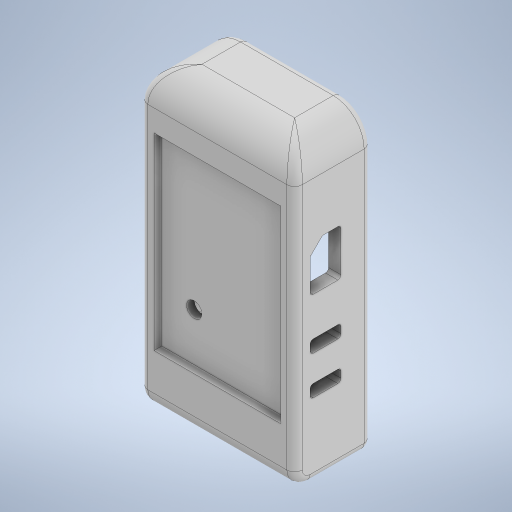
# Autodesk Inventor part: Součást1
Saved by Autodesk Inventor 2024 (Build 280153000, 153)
## iProperties
Created: 2024-02-27
Part Number: Součást1
Material: Všeobecné
Document SubType Name: Modeling
Designer: zak
Density: 1 g/cm^3
Appearance: Výchozí
Author: zak
Autodesk Inventor part; units mm, degrees
ref_plane "YZ Plane" through (0, 0, 0) normal (1, 0, 0) x (0, 1, 0)
ref_plane "XZ Plane" through (0, 0, 0) normal (0, 1, 0) x (-1, 0, 0)
ref_plane "XY Plane" through (0, 0, 0) normal (0, 0, 1) x (1, 0, 0)
sketch "Náčrt1" plane through (0, 0, 0) normal (0, 0, 1) x (1, 0, 0)
  line L0 (-50, -95) -> (50, -95)
  line L1 (50, -95) -> (50, 95)
  line L2 (50, 95) -> (-50, 95)
  line L3 (-50, 95) -> (-50, -95)
  line L4 (-50, -95) -> (50, 95) construction
  line L5 (50, -95) -> (-50, 95) construction
  point P0 (0, 0)
  dimension "d0" = 100
  dimension "d1" = 190
  constraints: 12 end point, 2 midpoint, 2 parallel, 1 horizontal, 1 perpendicular
  measures "d0" distance of L2.end L1.end
  measures "d1" distance of L1.end L0.end
extrude "Vysunutí1" add sketch "Náčrt1" along normal blind 50
sketch "Náčrt2" plane through (0, 0, 0) normal (0, 0, -1) x (-1, 0, 0)
  point P0 (0, 0)
sketch "Náčrt4" plane through (0, 0, 0) normal (0, 0, -1) x (-1, 0, 0)
  line L0 (42, 45) -> (-42, 45)
  line L1 (-42, 45) -> (-42, -65)
  line L2 (-42, -65) -> (42, -65)
  line L3 (42, -65) -> (42, 45)
  line L4 (42, 45) -> (-42, -65) construction
  line L5 (-42, 45) -> (42, -65) construction
  point P0 (0, 0)
  point P1 (0, -10)
  dimension "d8" = 84
  dimension "d9" = 110
  constraints: 12 end point, 2 midpoint, 2 parallel, 1 horizontal, 1 perpendicular
  measures "d8" distance of L2.end L1.end
  measures "d9" distance of L1.end L0.end
extrude "Vysunutí3" cut sketch "Náčrt4" against normal blind 40
fillet "Zaoblení1" radius 20 3 edges at (0, 95, 50) (-50, 95, 25) (50, 95, 25)
fillet "Zaoblení2" radius 10 1 edges at (0, -95, 50)
sketch "Náčrt5" plane through (0, 0, 40) normal (0, 0, -1) x (-1, 0, 0)
  circle A0 centre (37, 40) radius 5
  line L0 (42, 45) -> (42, -65) projected
  line L1 (-42, 45) -> (42, 45) projected
  circle A1 centre (37, -60) radius 5
  circle A2 centre (-37, 40) radius 5
  circle A3 centre (-37, -60) radius 5
  line L2 (42, 45) -> (32, 45)
  line L3 (32, 45) -> (32, 35)
  line L4 (32, 35) -> (42, 35)
  line L5 (42, 35) -> (42, 45)
  line L6 (42, 45) -> (32, 35) construction
  line L7 (32, 45) -> (42, 35) construction
  line L8 (42, -65) -> (32, -65)
  line L9 (32, -65) -> (32, -55)
  line L10 (32, -55) -> (42, -55)
  line L11 (42, -55) -> (42, -65)
  line L12 (42, -65) -> (32, -55) construction
  line L13 (32, -65) -> (42, -55) construction
  line L14 (-42, -65) -> (-32, -65)
  line L15 (-32, -65) -> (-32, -55)
  line L16 (-32, -55) -> (-42, -55)
  line L17 (-42, -55) -> (-42, -65)
  line L18 (-42, -65) -> (-32, -55) construction
  line L19 (-32, -65) -> (-42, -55) construction
  line L20 (-32, 45) -> (-42, 45)
  line L21 (-42, 45) -> (-42, 35)
  line L22 (-42, 35) -> (-32, 35)
  line L23 (-32, 35) -> (-32, 45)
  line L24 (-32, 45) -> (-42, 35) construction
  line L25 (-42, 45) -> (-32, 35) construction
  line L26 (42, 45) -> (32, 45)
  line L27 (32, 45) -> (32, 35)
  line L28 (32, 35) -> (42, 35)
  line L29 (42, 35) -> (42, 45)
  line L30 (42, 45) -> (32, 35) construction
  line L31 (32, 45) -> (42, 35) construction
  line L32 (32, -55) -> (32, -65)
  line L33 (32, -65) -> (42, -65)
  line L34 (42, -65) -> (42, -55)
  line L35 (42, -55) -> (32, -55)
  line L36 (-42, 45) -> (-42, 35)
  line L37 (-42, 35) -> (-32, 35)
  line L38 (-32, 35) -> (-32, 45)
  line L39 (-32, 45) -> (-42, 45)
  line L40 (-42, -55) -> (-42, -65)
  line L41 (-42, -65) -> (-32, -65)
  line L42 (-32, -65) -> (-32, -55)
  line L43 (-32, -55) -> (-42, -55)
  point P0 (0, 0)
  point P1 (32, -155)
  point P2 (-116, 35)
  point P3 (-42, -155)
  point P4 (-116, -65)
  point P5 (-32, 40)
  point P6 (-37, 35)
  point P7 (-37, 45)
  point P8 (-42, 40)
  point P9 (-42, -60)
  point P10 (-37, -55)
  point P11 (-37, -65)
  point P12 (-32, -60)
  point P13 (37, -65)
  point P14 (42, -60)
  point P15 (32, -60)
  point P16 (37, -55)
  point P17 (37, 45)
  point P18 (42, 40)
  point P19 (32, 40)
  point P20 (37, 35)
  dimension "d16" = 100
  dimension "d19" = 74
  dimension "d143" = 100
  dimension "d146" = 74
  constraints: 84 end point, 10 midpoint, 10 parallel, 10 point on line, 7 horizontal, 5 perpendicular, 4 centre point, 2 vertical, 1 tangent, 36 other
  measures "d16" distance of A0.centre A1.centre
  measures "d19" distance of A0.centre A2.centre
  measures "d143" distance of L2.end L32.start
  measures "d146" distance of L2.end L36.start
extrude "Vysunutí4" add sketch "Náčrt5" along normal blind 40
sketch "Náčrt6" plane through (0, 0, 0) normal (0, 0, -1) x (-1, 0, 0)
  arc A0 (37, 45) -> (42, 40) centre (37, 40) ccw projected
  circle A1 centre (37, 40) radius 2.5
  circle A2 centre (-37, 40) radius 2.5
  arc A3 (-37, -65) -> (-42, -60) centre (-37, -60) ccw projected
  circle A4 centre (-37, -60) radius 2.5
  arc A5 (42, -60) -> (37, -65) centre (37, -60) ccw projected
  circle A6 centre (37, -60) radius 2.5
  point P0 (0, 0)
  dimension "d24" = 5
  dimension "d25" = 5
  dimension "d26" = 5
  dimension "d27" = 5
  constraints: 4 centre point, 3 coincident
  measures "d24" diameter of A1
  measures "d25" diameter of A2
  measures "d26" diameter of A4
  measures "d27" diameter of A6
extrude "Vysunutí5" cut sketch "Náčrt6" against normal blind 10
sketch "Náčrt9" plane through (-37, -65, 0) normal (0, 1, 0) x (1, 0, 0)
  line L0 (30.5, -29) -> (43.5, -29)
  line L1 (43.5, -29) -> (43.5, -11)
  line L2 (43.5, -11) -> (30.5, -11)
  line L3 (30.5, -11) -> (30.5, -29)
  line L4 (30.5, -29) -> (43.5, -11) construction
  line L5 (43.5, -29) -> (30.5, -11) construction
  circle A0 centre (30.5, -11) radius 1.75
  circle A1 centre (43.5, -11) radius 1.75
  circle A2 centre (43.5, -29) radius 1.75
  circle A3 centre (30.5, -29) radius 1.75
  circle A4 centre (30.5, -29) radius 1
  circle A5 centre (30.5, -11) radius 1
  circle A6 centre (43.5, -11) radius 1
  circle A7 centre (43.5, -29) radius 1
  point P0 (37, 0)
  point P1 (37, -20)
  dimension "d30" = 13
  dimension "d31" = 18
  dimension "d32" = 3.5
  dimension "d33" = 3.5
  dimension "d34" = 3.5
  dimension "d35" = 3.5
  dimension "d128" = 2
  dimension "d129" = 2
  dimension "d130" = 2
  dimension "d131" = 2
  constraints: 12 end point, 8 centre point, 7 coincident, 2 midpoint, 2 parallel, 1 horizontal, 1 perpendicular, 1 point on line
  measures "d30" distance of L2.end L1.end
  measures "d31" distance of L1.end L0.end
  measures "d32" diameter of A0
  measures "d33" diameter of A1
  measures "d34" diameter of A2
  measures "d35" diameter of A3
  measures "d128" diameter of A4
  measures "d129" diameter of A5
  measures "d130" diameter of A6
  measures "d131" diameter of A7
extrude "Vysunutí6" add sketch "Náčrt9" along normal blind 4 contours A4 L3 A3 L0 | L0 A3 L3 A4 | A2 L1 A7 L0 | L0 A7 L1 A2 | A0 L2 A5 L3 | L3 A5 L2 A0 | A1 L2 A6 L1 | L1 A6 L2 A1
sketch "Náčrt11" plane through (-37, 45, 0) normal (0, -1, 0) x (1, 0, 0)
  line L0 (30.5, 11) -> (43.5, 11)
  line L1 (43.5, 11) -> (43.5, 29)
  line L2 (43.5, 29) -> (30.5, 29)
  line L3 (30.5, 29) -> (30.5, 11)
  line L4 (30.5, 11) -> (43.5, 29) construction
  line L5 (43.5, 11) -> (30.5, 29) construction
  circle A0 centre (30.5, 11) radius 1.75
  circle A1 centre (30.5, 29) radius 1.75
  circle A2 centre (43.5, 11) radius 1.75
  circle A3 centre (43.5, 29) radius 1.75
  circle A4 centre (30.5, 11) radius 1
  circle A5 centre (30.5, 29) radius 1
  circle A6 centre (43.5, 11) radius 1
  circle A7 centre (43.5, 29) radius 1
  point P0 (37, 0)
  point P1 (37, 20)
  dimension "d49" = 13
  dimension "d50" = 18
  dimension "d51" = 3.5
  dimension "d52" = 3.5
  dimension "d53" = 3.5
  dimension "d54" = 3.5
  dimension "d132" = 2
  dimension "d135" = 18
  dimension "d138" = 13
  constraints: 12 end point, 8 centre point, 5 coincident, 2 horizontal, 2 midpoint, 2 parallel, 1 perpendicular, 1 vertical, 6 other
  measures "d49" distance of L2.end L1.end
  measures "d50" distance of L1.end L0.end
  measures "d51" diameter of A0
  measures "d52" diameter of A1
  measures "d53" diameter of A2
  measures "d54" diameter of A3
  measures "d132" diameter of A4
  measures "d135" distance of A4.centre A5.centre
  measures "d138" distance of A4.centre A6.centre
extrude "Vysunutí8" add sketch "Náčrt11" along normal blind 4 contours A4 L3 A0 L0 | L0 A0 L3 A4 | A2 L1 A6 L0 | L0 A6 L1 A2 | A1 L2 A5 L3 | L3 A5 L2 A1 | A3 L2 A7 L1 | L1 A7 L2 A3
fillet "Zaoblení3" radius 5 8 edges at (-50, -92.0711, 47.0711) (-50, -95, 20) (-44.1421, 89.1421, 44.1421) (-50, -5, 50) (44.1421, 89.1421, 44.1421) (50, -92.0711, 47.0711) (50, -95, 20) (50, -5, 50)
fillet "Zaoblení4" radius 5 8 edges at (-44.1421, 89.1421, 0) (-50, -7.5, 0) (-48.5355, -93.5355, 0) (0, -95, 0) (48.5355, -93.5355, 0) (50, -7.5, 0) (44.1421, 89.1421, 0) (0, 95, 0)
sketch "Náčrt17" plane through (0, 0, 0) normal (0, 0, -1) x (-1, 0, 0)
  line L0 (38.0929, 83.7446) -> (-38.0929, 83.7446)
  line L1 (-40.0929, 81.7446) -> (-40.0929, 58.2554)
  line L2 (-38.0929, 56.2554) -> (38.0929, 56.2554)
  line L3 (40.0929, 58.2554) -> (40.0929, 81.7446)
  line L4 (40.0929, 83.7446) -> (-40.0929, 56.2554) construction
  line L5 (-40.0929, 83.7446) -> (40.0929, 56.2554) construction
  arc A0 (40.0929, 81.7446) -> (38.0929, 83.7446) centre (38.0929, 81.7446) ccw
  arc A1 (38.0929, 56.2554) -> (40.0929, 58.2554) centre (38.0929, 58.2554) ccw
  arc A2 (-40.0929, 58.2554) -> (-38.0929, 56.2554) centre (-38.0929, 58.2554) ccw
  arc A3 (-38.0929, 83.7446) -> (-40.0929, 81.7446) centre (-38.0929, 81.7446) ccw
  line L6 (40, -87.5) -> (-40, -87.5)
  line L7 (-42, -85.5) -> (-42, -74.5)
  line L8 (-40, -72.5) -> (40, -72.5)
  line L9 (42, -74.5) -> (42, -85.5)
  line L10 (42, -87.5) -> (-42, -72.5) construction
  line L11 (-42, -87.5) -> (42, -72.5) construction
  arc A4 (40, -87.5) -> (42, -85.5) centre (40, -85.5) ccw
  arc A5 (42, -74.5) -> (40, -72.5) centre (40, -74.5) ccw
  arc A6 (-40, -72.5) -> (-42, -74.5) centre (-40, -74.5) ccw
  arc A7 (-42, -85.5) -> (-40, -87.5) centre (-40, -85.5) ccw
  point P0 (0, 0)
  point P1 (0, 70)
  point P2 (0, -80)
  dimension "d82" = 2
  dimension "d83" = 15
  dimension "d84" = 2
  constraints: 24 end point, 16 point on circle, 16 point on line, 16 tangent, 8 centre point, 6 equal radius, 4 midpoint, 4 parallel, 2 horizontal, 2 perpendicular
  measures "d82" radius of A0
  measures "d83" distance of L11.start L10.end
  measures "d84" radius of A4
extrude "Vysunutí12" cut sketch "Náčrt17" against normal blind 35
sketch "Náčrt18" plane through (0, 0, 50) normal (0, 0, 1) x (1, 0, 0)
  line L0 (41, 61) -> (-41, 61)
  line L1 (-41, 61) -> (-41, -61)
  line L2 (-41, -61) -> (41, -61)
  line L3 (41, -61) -> (41, 61)
  line L4 (41, 61) -> (-41, -61) construction
  line L5 (-41, 61) -> (41, -61) construction
  point P0 (0, 0)
  dimension "d87" = 82
  dimension "d88" = 122
  constraints: 12 end point, 2 midpoint, 2 parallel, 1 horizontal, 1 perpendicular
  measures "d87" distance of L2.end L1.end
  measures "d88" distance of L1.end L0.end
extrude "Vysunutí13" cut sketch "Náčrt18" against normal blind 5
sketch "Náčrt20" plane through (-50, -85, 45) normal (-1, 0, 0) x (0, 0, 1)
  line L0 (-5, 120) -> (-5, 30) projected
  line L1 (-13.8284, 125) -> (-23, 125)
  line L2 (-25, 123) -> (-25, 97)
  line L3 (-23, 95) -> (-7, 95)
  line L4 (-5, 97) -> (-5, 116.1716)
  line L5 (-5.5858, 117.5858) -> (-12.4142, 124.4142)
  arc A0 (-23, 125) -> (-25, 123) centre (-23, 123) ccw
  arc A1 (-12.4142, 124.4142) -> (-13.8284, 125) centre (-13.8284, 123) ccw
  arc A2 (-5, 116.1716) -> (-5.5858, 117.5858) centre (-7, 116.1716) ccw
  arc A3 (-7, 95) -> (-5, 97) centre (-7, 97) ccw
  arc A4 (-25, 97) -> (-23, 95) centre (-23, 97) ccw
  line L6 (-7, 70) -> (-23, 70)
  line L7 (-25, 68) -> (-25, 64)
  line L8 (-23, 62) -> (-7, 62)
  line L9 (-5, 64) -> (-5, 68)
  line L10 (-7, 45) -> (-23, 45)
  line L11 (-25, 43) -> (-25, 39)
  line L12 (-23, 37) -> (-7, 37)
  line L13 (-5, 39) -> (-5, 43)
  arc A5 (-5, 68) -> (-7, 70) centre (-7, 68) ccw
  arc A6 (-7, 62) -> (-5, 64) centre (-7, 64) ccw
  arc A7 (-23, 70) -> (-25, 68) centre (-23, 68) ccw
  arc A8 (-25, 64) -> (-23, 62) centre (-23, 64) ccw
  arc A9 (-23, 45) -> (-25, 43) centre (-23, 43) ccw
  arc A10 (-5, 43) -> (-7, 45) centre (-7, 43) ccw
  arc A11 (-7, 37) -> (-5, 39) centre (-7, 39) ccw
  arc A12 (-25, 39) -> (-23, 37) centre (-23, 39) ccw
  point P0 (-45, 85)
  point P1 (-5, 125)
  point P2 (-5, 25)
  point P3 (-25, 95)
  point P4 (-25, 125)
  point P5 (-5, 95)
  point P6 (-5, 117)
  point P7 (-13, 125)
  point P8 (-25, 62)
  point P9 (-25, 70)
  point P10 (-5, 62)
  point P11 (-5, 45)
  point P12 (-25, 37)
  point P13 (-25, 45)
  point P14 (-5, 37)
  point P15 (-5, 97)
  dimension "d94" = 20
  dimension "d95" = 30
  dimension "d96" = 8
  dimension "d97" = 8
  dimension "d98" = 2
  dimension "d99" = 20
  dimension "d100" = 8
  dimension "d101" = 20
  dimension "d102" = 8
  dimension "d103" = 2
  constraints: 27 point on line, 26 end point, 26 point on circle, 26 tangent, 13 centre point, 11 equal radius, 6 parallel, 3 horizontal, 3 perpendicular
  measures "d94" distance of point (-5, 95) point (-25, 95)
  measures "d95" distance of point (-25, 95) point (-25, 125)
  measures "d96" distance of point (-5, 117) point (-5, 125)
  measures "d97" distance of point (-13, 125) point (-5, 125)
  measures "d98" radius of A0
  measures "d99" distance of point (-5, 62) point (-25, 62)
  measures "d100" distance of point (-25, 62) point (-25, 70)
  measures "d101" distance of point (-5, 37) point (-25, 37)
  measures "d102" distance of point (-25, 37) point (-25, 45)
  measures "d103" radius of A5
extrude "Vysunutí15" cut sketch "Náčrt20" against normal blind 100
sketch "Náčrt21" plane through (0, 0, 40) normal (0, 0, -1) x (-1, 0, 0)
  line L0 (-5.5, 23.5) -> (5.5, 23.5)
  line L1 (5.5, 23.5) -> (5.5, -23.5)
  line L2 (5.5, -23.5) -> (-5.5, -23.5)
  line L3 (-5.5, -23.5) -> (-5.5, 23.5)
  line L4 (-5.5, 23.5) -> (5.5, -23.5) construction
  line L5 (5.5, 23.5) -> (-5.5, -23.5) construction
  circle A0 centre (5.5, 23.5) radius 1.75
  circle A1 centre (-5.5, 23.5) radius 1.75
  circle A2 centre (5.5, -23.5) radius 1.75
  circle A3 centre (-5.5, -23.5) radius 1.75
  circle A4 centre (-5.5, 23.5) radius 1
  circle A5 centre (5.5, 23.5) radius 1
  circle A6 centre (-5.5, -23.5) radius 1
  circle A7 centre (5.5, -23.5) radius 1
  point P0 (0, 0)
  dimension "d106" = 11
  dimension "d107" = 47
  dimension "d108" = 3.5
  dimension "d111" = 11
  dimension "d114" = 47
  dimension "d117" = 2
  dimension "d120" = 11
  dimension "d123" = 47
  constraints: 12 end point, 8 centre point, 3 horizontal, 2 coincident, 2 midpoint, 2 parallel, 2 vertical, 1 perpendicular, 12 other
  measures "d106" distance of L1.end L2.end
  measures "d107" distance of L0.end L1.end
  measures "d108" diameter of A0
  measures "d111" distance of A0.centre A1.centre
  measures "d114" distance of A0.centre A2.centre
  measures "d117" diameter of A4
  measures "d120" distance of A4.centre A5.centre
  measures "d123" distance of A4.centre A6.centre
extrude "Vysunutí16" add sketch "Náčrt21" along normal blind 5 contours A4 L3 A1 L0 | L0 A1 L3 A4 | A0 L1 A5 L0 | L0 A5 L1 A0 | A3 L2 A6 L3 | L3 A6 L2 A3 | A2 L2 A7 L1 | L1 A7 L2 A2
sketch "Náčrt25" plane through (0, 0, 45) normal (0, 0, 1) x (1, 0, 0)
  circle A0 centre (-20, -30) radius 5
  point P0 (0, 0)
  dimension "d149" = 10
  constraints: 1 centre point
  measures "d149" diameter of A0
extrude "Vysunutí17" cut sketch "Náčrt25" against normal blind 10
sketch "Náčrt26" plane through (-32, -65, 0) normal (0, 1, 0) x (1, 0, 0)
  circle A0 centre (55, -20) radius 6
  point P0 (32, 0)
  dimension "d152" = 12
  constraints: 1 centre point
  measures "d152" diameter of A0
extrude "Vysunutí18" cut sketch "Náčrt26" against normal blind 100
equation "\"d97\" = d96"
